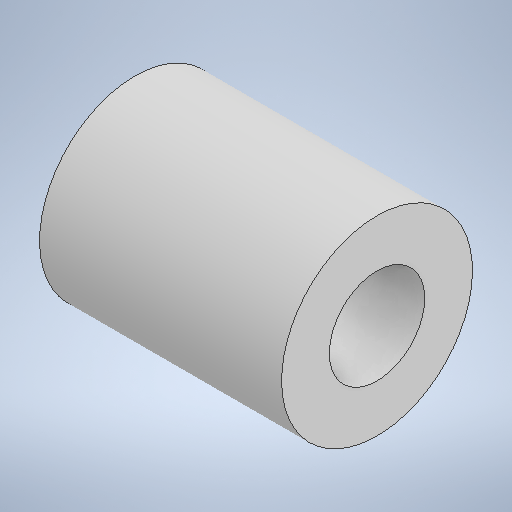
# Autodesk Inventor part: Part1
Saved by Autodesk Inventor 2025.2 (Build 292293000, 293)
## iProperties
Created: 2026-03-09
Part Number: Part1
Material: Generic
Document SubType Name: Modeling
Designer: Simon
Density: 1 g/cm^3
Appearance: Default
Author: Simon
Autodesk Inventor part; units mm, degrees
ref_plane "YZ Plane" through (0, 0, 0) normal (1, 0, 0) x (0, 1, 0)
ref_plane "XZ Plane" through (0, 0, 0) normal (0, 1, 0) x (-1, 0, 0)
ref_plane "XY Plane" through (0, 0, 0) normal (0, 0, 1) x (1, 0, 0)
sketch "Sketch1" plane through (0, 0, 0) normal (0, 0, 1) x (1, 0, 0)
  line L0 (0, 0) -> (0, 2)
  line L1 (0, 2) -> (50, 2)
  line L2 (0, 0) -> (0, 0.1)
  line L3 (0, 0.1) -> (50, 0.1)
  line L4 (0, 0) -> (0, 5)
  line L5 (0, 5) -> (50, 5)
  line L6 (0, 0) -> (0, 4)
  line L7 (0, 4) -> (4, 4)
  line L8 (4, 4) -> (4, 2)
  line L9 (4, 2) -> (4, 10)
  line L10 (4, 2) -> (6.7109, 2) construction
  line L11 (4, 10) -> (7, 10)
  line L12 (7, 10) -> (7, 2)
  line L13 (7, 2) -> (14.0909, 0.1)
  line L14 (7, 2) -> (9.25, 2) construction
  line L15 (14.0909, 0.1) -> (32.3779, 5)
  line L16 (14.0909, 0.1) -> (33.023, 0.1) construction
  line L17 (32.3779, 5) -> (32.3779, 7)
  line L18 (32.3779, 7) -> (7, 10)
  line L19 (0, 0) -> (50, 0)
  line L20 (-10, 0) -> (60, 0) projected
  line L21 (32.3779, 7) -> (32.3779, 10)
  line L22 (32.3779, 10) -> (7, 10)
  point P0 (0, 2)
  point P1 (7, 5)
  point P2 (4, 5)
  point P3 (17.0086, 2)
  point P4 (21.1818, 2)
  dimension "d0" = 2
  dimension "d1" = 50
  dimension "d2" = 0.1
  dimension "d3" = 5
  dimension "d4" = 4
  dimension "d5" = 4
  dimension "d6" = 8
  dimension "d8" = 3
  dimension "d9" = 15
  dimension "d10" = 15
  dimension "d13" = 50
  constraints: 44 end point, 7 perpendicular, 7 point on line, 5 horizontal, 3 vertical, 1 collinear, 1 equal length
  measures "d0" distance of L0.start L0.end
  measures "d1" distance of L0.end L1.end
  measures "d2" distance of L0.start L2.end
  measures "d3" distance of L0.start L4.end
  measures "d4" distance of L0.start L6.end
  measures "d5" distance of L6.end L7.end
  measures "d6" distance of L8.end L9.end
  measures "d8" distance of L9.end L11.end
  measures "d9" angle of L13 L14
  measures "d10" angle of L16 L15
  measures "d13" distance of L0.start L19.end
revolve "Revolution2" add sketch "Sketch1" angle 360 about axis through (-10, 0, 0) along (1, 0, 0) contours L13 L1 L15 | L12 L5 L15 L1 | L12 L18 L17 L5 | L22 L21 L18
body "Solid2"
